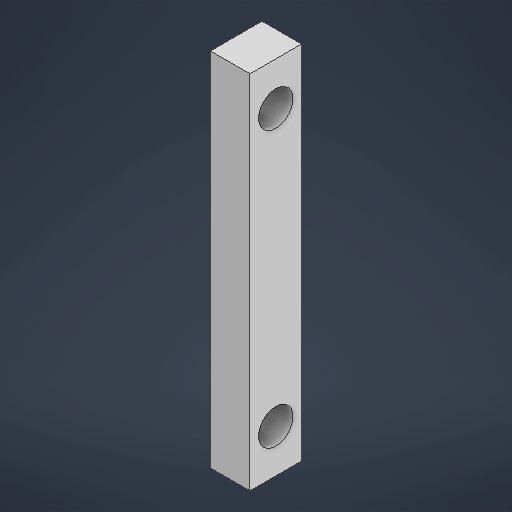
# Autodesk Inventor part: BearingBlockSpacer
Saved by Autodesk Inventor 2025 (Build 290162000, 162)
## iProperties
Created: 2024-05-20
Part Number: BearingBlockSpacer
Material: Generic
Document SubType Name: Modeling
Designer: avsar
Density: 1 g/cm^3
Appearance: Default
Author: avsar
Autodesk Inventor part; units mm, degrees
ref_plane "YZ Plane" through (0, 0, 0) normal (1, 0, 0) x (0, 1, 0)
ref_plane "XZ Plane" through (0, 0, 0) normal (0, 1, 0) x (-1, 0, 0)
ref_plane "XY Plane" through (0, 0, 0) normal (0, 0, 1) x (1, 0, 0)
sketch "Sketch1" plane through (0, 0, 0) normal (1, 0, 0) x (0, 1, 0)
  circle A0 centre (16, 0) radius 2
  circle A1 centre (-16, 0) radius 2
  line L0 (-21, 3) -> (21, 3)
  line L1 (21, 3) -> (21, -3)
  line L2 (21, -3) -> (-21, -3)
  line L3 (-21, -3) -> (-21, 3)
  line L4 (-21, 3) -> (21, -3) construction
  line L5 (21, 3) -> (-21, -3) construction
  point P0 (0, 0)
  dimension "d0" = 16
  dimension "d1" = 16
  dimension "d2" = 42
  dimension "d3" = 4
  dimension "d4" = 4
  dimension "d5" = 6
  constraints: 12 end point, 2 centre point, 2 horizontal alignment, 2 midpoint, 2 parallel, 1 horizontal, 1 perpendicular
  measures "d0" distance of point (0, 0) A0.centre
  measures "d1" distance of A1.centre point (0, 0)
  measures "d2" distance of L1.end L2.end
  measures "d3" diameter of A0
  measures "d4" diameter of A1
  measures "d5" distance of L0.end L1.end
extrude "Extrusion1" add sketch "Sketch1" along normal blind 4.6
body "Solid1"
